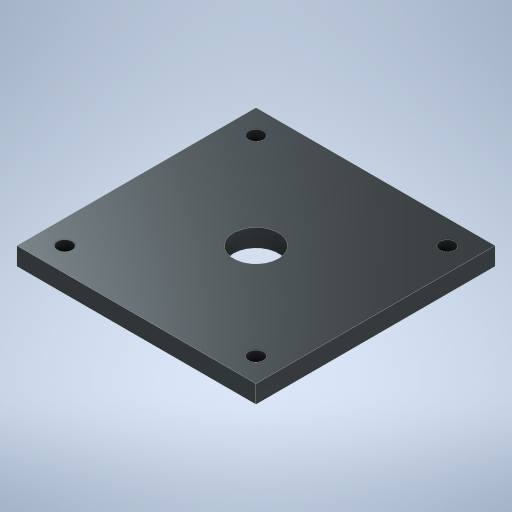
# Autodesk Inventor part: Suporte inferior do eixo
Saved by Autodesk Inventor 2023 (Build 270158000, 158)
## iProperties
Created: 2023-03-21
Part Number: Suporte inferior do eixo
Material: Aluminum 6061
Document SubType Name: Sheet Metal
Designer: Mateus PC
Density: 2.7 g/cm^3
Sheet Metal Rule: Default_mm
Appearance: Ferro cinza
Mass: 100.257 g
Surface Area: 149.195 cm^2
Volume: 37.1324 cm^3
Author: Mateus
Autodesk Inventor part; units mm, degrees
ref_plane "YZ Plane" through (0, 0, 0) normal (1, 0, 0) x (0, 1, 0)
ref_plane "XZ Plane" through (0, 0, 0) normal (0, 1, 0) x (-1, 0, 0)
ref_plane "XY Plane" through (0, 0, 0) normal (0, 0, 1) x (1, 0, 0)
sketch "Esboço1" plane through (0, 0, 0) normal (0, 1, 0) x (-1, 0, 0)
  line L0 (0, 0) -> (80, 0)
  line L1 (80, 0) -> (80, -80)
  line L2 (80, -80) -> (0, -80)
  line L3 (0, -80) -> (0, 0)
  dimension "d0" = 80
  dimension "d1" = 80
  constraints: 8 end point, 2 parallel, 1 horizontal, 1 perpendicular
  measures "d0" distance of L0.end L1.end
  measures "d1" distance of L1.end L2.end
extrude "Extrusão1" add sketch "Esboço1" along normal blind 6
sketch "Esboço2" plane through (0, 6, 0) normal (0, 1, 0) x (1, 0, 0)
  line L0 (0, 80) -> (-80, 80) projected
  line L1 (-80, 80) -> (-80, 0) projected
  line L2 (-80, 0) -> (0, 0) projected
  line L3 (0, 0) -> (0, 80) projected
  point P0 (-8, 8)
  point P1 (-72, 8)
  point P2 (-72, 72)
  point P3 (-8, 72)
  dimension "d4" = 8
  dimension "d5" = 8
  dimension "d6" = 8
  dimension "d7" = 8
  dimension "d8" = 8
  dimension "d9" = 8
  dimension "d10" = 8
  dimension "d11" = 8
  measures "d4" distance from line of L0 point (-72, 72)
  measures "d5" distance from line of L1 point (-72, 72)
  measures "d6" distance from line of L1 point (-72, 8)
  measures "d7" distance from line of L2 point (-72, 8)
  measures "d8" distance from line of L2 point (-8, 8)
  measures "d9" distance from line of L3 point (-8, 8)
  measures "d10" distance from line of L3 point (-8, 72)
  measures "d11" distance from line of L0 point (-8, 72)
hole "Furo1" at (-8, 6, -8) at (-72, 6, -8) at (-72, 6, -72) at (-8, 6, -72) direction (0, -1, 0) diameter 5 depth 6
sketch "Esboço3" plane through (0, 6, 0) normal (0, 1, 0) x (1, 0, 0)
  line L0 (-80, 0) -> (0, 0) projected
  line L1 (-80, 80) -> (-80, 0) projected
  line L2 (0, 80) -> (-80, 80) projected
  line L3 (0, 0) -> (0, 80) projected
  point P0 (-40, 40)
  dimension "d19" = 80
  dimension "d20" = 40
  dimension "d21" = 40
  measures "d19" distance of L1.start L0.start
  measures "d20" distance from line of L2 point (-40, 40)
  measures "d21" distance from line of L3 point (-40, 40)
hole "Furo2" at (-40, 6, -40) direction (0, -1, 0) diameter 15 depth 6
equation "\"d5\" = d4"
equation "\"d6\" = d5"
equation "\"d7\" = d5"
equation "\"d8\" = d7"
equation "\"d9\" = d6"
equation "\"d10\" = d9"
equation "\"d11\" = d4"
equation "\"d17\" = Espessura"
equation "\"d20\" = 0.5 * d19"
equation "\"d21\" = 0.5 * d19"
equation "\"Raio_vergadura\" = Espessura"
equation "\"Largura_alívio_de_vergadura\" = Espessura"
equation "\"Profundidade_alívio_de_vergadura\" = 0.5 * Espessura"
equation "\"Tamanho_alívio_de_dobra\" = 4 * Espessura"
equation "\"Remanescente_mínimo\" = 2 * Espessura"
equation "\"Raiodetransição\" = Raio_vergadura"
equation "\"Tamanho_de_raio_de_Jacobi\" = Raio_vergadura"
equation "\"TamanhoFolga\" = Espessura"
equation "\"Espessura\" = 0.5"
